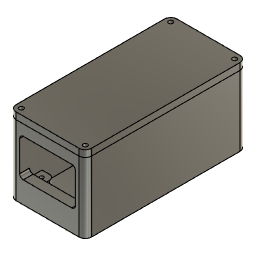
smarter-ac-unit (Autodesk Fusion 360 design; units mm, degrees)
Autodesk Fusion 360 part; units mm, degrees
sketch "top" plane through (0, 0, 0) normal (0, 0, 1) x (1, 0, 0)
  line L0 (0, 0) -> (31, 0)
  line L1 (31, 0) -> (31, 78.5)
  line L2 (31, 78.5) -> (0, 78.5)
  line L3 (0, 78.5) -> (0, 0)
  line L4 (36.5, -5.5) -> (36.5, 84)
  line L5 (36.5, 84) -> (-5.5, 84)
  line L6 (-5.5, 84) -> (-5.5, -5.5)
  line L7 (-5.5, -5.5) -> (36.5, -5.5)
  line L8 (-5.5, 39.25) -> (36.5, 39.25) construction
  line L9 (15.5, -5.5) -> (15.5, 84) construction
  line L10 (-5.5, -5.5) -> (0, 0) construction
  circle A0 centre (-2.2804, -2.2804) radius 1.225
  line L11 (-5.5, 67) -> (36.5, 67)
  line L12 (-5.5, 61.5) -> (0, 61.5)
  circle A1 centre (3.375, 3.375) radius 2.125
  circle A2 centre (3.375, 75.125) radius 2.125
  circle A3 centre (27.625, 3.375) radius 2.125
  circle A4 centre (27.625, 75.125) radius 2.125
  circle A5 centre (-2.2804, 80.7804) radius 1.225
  circle A6 centre (33.2804, -2.2804) radius 1.225
  circle A7 centre (33.2804, 80.7804) radius 1.225
  circle A8 centre (3.375, 3.375) radius 1
  circle A9 centre (27.625, 3.375) radius 1
  circle A10 centre (27.625, 75.125) radius 1
  circle A11 centre (3.375, 75.125) radius 1
  line L13 (0, 7) -> (7, 7)
  line L14 (7, 7) -> (7, 0)
  line L15 (24, 7) -> (24, 0)
  line L16 (31, 7) -> (24, 7)
  line L17 (24, 71.5) -> (24, 78.5)
  line L18 (31, 71.5) -> (24, 71.5)
  line L19 (7, 71.5) -> (7, 78.5)
  line L20 (0, 71.5) -> (7, 71.5)
  point P0 (-2.2804, -2.2804)
  dimension "d1" = 31
  dimension "d2" = 78.5
  dimension "d3" = 5.5
  dimension "d4" = 2.45
  dimension "d5" = 17
  dimension "d6" = 5.5
  dimension "d7" = 4.25
  dimension "d8" = 1.25
  dimension "d9" = 1.25
  dimension "d10" = 2
  dimension "d41" = 2
  dimension "d45" = 7
  dimension "d46" = 7
  constraint horizontal L0
  constraint vertical L1
  constraint horizontal L2
  constraint vertical L3
  constraint coincident L0.start L3.end
  constraint midpoint L6 L8.start
  constraint midpoint L4 L8.end
  constraint midpoint L7 L9.start
  constraint midpoint L5 L9.end
  constraint coincident P0 A0.centre
  constraint coincident L6 L11.start
  constraint coincident L4 L11.end
  constraint perpendicular L4 L11
  constraint coincident L6 L12.start
  constraint coincident L3 L12.end
  constraint perpendicular L3 L12
  constraint symmetric L8 A1 A2
  constraint symmetric L9 A1 A3
  constraint symmetric L9 A2 A4
  constraint coincident L10 P0
  constraint symmetric L8 A0 A5
  constraint symmetric L9 A0 A6
  constraint symmetric L9 A5 A7
  constraint concentric A1 A8
  constraint symmetric L9 A8 A9
  constraint symmetric L8 A8 A11
  constraint symmetric L8 A9 A10
  constraint coincident L3 L13.start
  constraint perpendicular L3 L13
  constraint coincident L0 L14.end
  constraint perpendicular L0 L14
  constraint symmetric L9 L13.start L16.start
  constraint symmetric L9 L13.end L15.start
  constraint symmetric L9 L14.end L15.end
  constraint symmetric L8 L13.start L20.start
  constraint symmetric L8 L13.end L19.start
  constraint symmetric L8 L14.end L19.end
  constraint symmetric L8 L15.start L17.start
  constraint symmetric L8 L15.end L17.end
  constraint symmetric L8 L16.start L18.start
  measures "d1" distance of L0.start L0.end
  measures "d2" distance of L0.start L2.end
  measures "d4" diameter of A0
  measures "d5" distance of L5 L11
  measures "d6" distance of L11 L12
  measures "d7" diameter of A1
  measures "d8" distance of L3 A1
  measures "d9" distance of L0 A1
  measures "d10" distance of L0.start A0
  measures "d41" diameter of A8
  measures "d45" distance of L13.start L13.end
  measures "d46" distance of L0 L13
extrude "Extrude1" add sketch "top" along normal blind 3 contours L0 L3 L13 L14 | L0 L1 L3 L4 L6 L7 L11 L12 | L0 L1 L3 L11 L13 L14 L15 L16 | L0 L1 L15 L16 | L3 L6 L11 L12 | L1 L2 L3 L4 L5 L6 L11 | L1 L2 L3 L11 L17 L18 L19 L20 | L2 L3 L19 L20 | L1 L2 L17 L18 | A0 | A1 | A2 | A3 | A4 | A5 | A6 | A7 | A8 | A9 | A10 | A11 makes body 1
extrude "Extrude2" add sketch "top" along normal blind 36 from surface at 3 contours L0 L1 L3 L4 L6 L7 L11 L12 | L3 L6 L11 L12 | L1 L2 L3 L4 L5 L6 L11 | A0 | A5 | A6 | A7 bodies 1
extrude "Extrude3" add sketch "top" along normal blind 6.5 from surface at 3 contours A1 | A2 | A3 | A4 | A8 | A9 | A10 | A11 bodies 1
sketch "side" plane through (-5.5, 0, 0) normal (-1, 0, 0) x (0, -1, 0)
  line L0 (-84, 0) -> (5.5, 0)
  line L1 (5.5, 0) -> (5.5, 39)
  line L2 (5.5, 39) -> (-84, 39)
  line L3 (-84, 39) -> (-84, 0)
  line L4 (-84, 0) -> (5.5, 0)
  line L5 (-84, 0) -> (-84, 39)
  line L6 (-84, 39) -> (5.5, 39)
  line L7 (5.5, 0) -> (5.5, 39)
  line L8 (-84, 19.5) -> (5.5, 19.5) construction
  line L9 (-1.25, 9.5) -> (-5.5, 9.5)
  line L10 (-73, 9.5) -> (-77.25, 9.5)
  line L11 (-5.5, 3) -> (-1.25, 3)
  line L12 (-77.25, 3) -> (-73, 3)
  line L13 (0, 3) -> (-78.5, 3)
  line L14 (0, 3) -> (0, 39)
  line L15 (-78.5, 3) -> (-78.5, 39)
  line L16 (-73, 9.5) -> (-5.5, 9.5) construction
  line L17 (-39.25, 39) -> (-39.25, 0) construction
  line L18 (-67, 0) -> (-67, 19.5) construction
  line L19 (-61.5, 0) -> (-61.5, 19.5) construction
  line L20 (-84, 14.5) -> (-61.5, 14.5) construction
  line L21 (-67, 14.5) -> (-61.5, 14.5)
  line L22 (-61.5, 14.5) -> (-61.5, 9.5)
  line L23 (-61.5, 9.5) -> (-67, 9.5)
  line L24 (-67, 9.5) -> (-67, 14.5)
  point P0 (-61.5, 0)
  point P1 (-67, 0)
  dimension "d19" = 5
  constraint midpoint L5 L8.start
  constraint midpoint L7 L8.end
  constraint coincident L10.start L16.start
  constraint coincident L9.end L16.end
  constraint midpoint L6 L17.start
  constraint midpoint L4 L17.end
  constraint coincident P1 L18.start
  constraint coincident L8 L18.end
  constraint perpendicular L8 L18
  constraint coincident P0 L19.start
  constraint coincident L8 L19.end
  constraint perpendicular L8 L19
  constraint coincident L5 L20.start
  constraint coincident L19 L20.end
  constraint perpendicular L19 L20
  constraint horizontal L21
  constraint vertical L22
  constraint horizontal L23
  constraint vertical L24
  constraint coincident L19 L22.end
  constraint coincident L16 L22.end
  constraint coincident L20 L21.start
  constraint coincident L18 L21.start
  measures "d19" distance of L16 L20
extrude "Extrude4" cut sketch "side" against normal up to surface (5.5 mm away) contours L21 L22 L23 L24 bodies 1
sketch "back" plane through (0, -5.5, 0) normal (0, -1, 0) x (1, 0, 0)
  line L0 (-5.5, 0) -> (36.5, 0)
  line L1 (36.5, 0) -> (36.5, 39)
  line L2 (36.5, 39) -> (-5.5, 39)
  line L3 (-5.5, 39) -> (-5.5, 0)
  line L4 (0, 3) -> (0, 39)
  line L5 (5.5, 9.5) -> (1.25, 9.5)
  line L6 (1.25, 3) -> (5.5, 3)
  line L7 (25.5, 3) -> (29.75, 3)
  line L8 (29.75, 9.5) -> (25.5, 9.5)
  line L9 (31, 3) -> (31, 39)
  line L10 (31, 3) -> (0, 3)
  line L11 (0, 39) -> (31, 39)
  line L12 (-5.5, 0) -> (36.5, 0)
  line L13 (36.5, 0) -> (36.5, 39)
  line L14 (-5.5, 0) -> (-5.5, 39)
  line L15 (0, 33) -> (31, 33)
  line L16 (0, 12) -> (31, 12)
  dimension "d22" = 6
  dimension "d23" = 2.5
  constraint coincident L4 L15.start
  constraint coincident L9 L15.end
  constraint perpendicular L9 L15
  constraint coincident L4 L16.start
  constraint coincident L9 L16.end
  constraint perpendicular L9 L16
  measures "d22" distance of L2 L15
  measures "d23" distance of L5 L16
extrude "Extrude5" cut sketch "back" against normal up to surface (5.5 mm away) contours L4 L9 L15 L16 bodies 1
sketch "front" plane through (0, 84, 0) normal (0, 1, 0) x (-1, 0, 0)
  line L0 (-36.5, 0) -> (5.5, 0)
  line L1 (5.5, 0) -> (5.5, 39)
  line L2 (5.5, 39) -> (-36.5, 39)
  line L3 (-36.5, 39) -> (-36.5, 0)
  line L4 (-36.5, 0) -> (-36.5, 39)
  line L5 (-36.5, 39) -> (5.5, 39)
  line L6 (5.5, 0) -> (5.5, 39)
  line L7 (-36.5, 0) -> (5.5, 0)
  line L8 (-25.5, 9.5) -> (-29.75, 9.5)
  line L9 (-1.25, 9.5) -> (-5.5, 9.5)
  line L10 (-31, 3) -> (0, 3)
  line L11 (0, 3) -> (0, 39)
  line L12 (-31, 3) -> (-31, 39)
  line L13 (-31, 12) -> (0, 12) construction
  line L14 (-15.5, 39) -> (-15.5, 12) construction
  circle A0 centre (-15.5, 12) radius 2.75
  dimension "d26" = 2.5
  dimension "d27" = 5.5
  constraint coincident L12 L13.start
  constraint coincident L11 L13.end
  constraint perpendicular L11 L13
  constraint midpoint L5 L14.start
  constraint midpoint L13 L14.end
  constraint coincident L14.end A0.centre
  measures "d26" distance of L8 L13
  measures "d27" diameter of A0
extrude "Extrude6" cut sketch "front" against normal up to surface (5.5 mm away) contours A0 bodies 1
extrude "Extrude7" cut sketch "top" against normal blind 5 from surface at 39 contours A0 | A5 | A6 | A7 bodies 1
sketch "lid" plane through (0, 0, 39) normal (0, 0, 1) x (-1, 0, 0)
  circle A0 centre (-33.2804, -80.7804) radius 1.225
  circle A1 centre (-33.2804, 2.2804) radius 1.225
  circle A2 centre (2.2804, -80.7804) radius 1.225
  circle A3 centre (2.2804, 2.2804) radius 1.225
  line L0 (-31, 0) -> (0, 0)
  line L1 (0, 0) -> (0, -78.5)
  line L2 (0, -78.5) -> (-31, -78.5)
  line L3 (-31, -78.5) -> (-31, 0)
  line L4 (5.5, -84) -> (5.5, 5.5)
  line L5 (5.5, 5.5) -> (-36.5, 5.5)
  line L6 (-36.5, 5.5) -> (-36.5, -84)
  line L7 (-36.5, -84) -> (5.5, -84)
  line L8 (5.5, -84) -> (5.5, 5.5)
  line L9 (-36.5, -84) -> (5.5, -84)
  line L10 (-36.5, 5.5) -> (-36.5, -84)
  line L11 (5.5, 5.5) -> (-36.5, 5.5)
  circle A4 centre (2.2804, 2.2804) radius 1.225
  circle A5 centre (-33.2804, 2.2804) radius 1.225
  circle A6 centre (-33.2804, -80.7804) radius 1.225
  circle A7 centre (2.2804, -80.7804) radius 1.225
  line L12 (0, 0) -> (0, -78.5)
  line L13 (0, -78.5) -> (-31, -78.5)
  line L14 (-31, -78.5) -> (-31, 0)
  line L15 (-31, 0) -> (0, 0)
extrude "Extrude8" add sketch "lid" along normal blind 3.75 separate body contours L0 L1 L2 L3 L12 L13 L14 L15 | L4 L5 L6 L7 L8 L9 L10 L11 makes body 2
fillet "Fillet1" radius 3.5 8 edges at (36.5, 84, 19.5) (-5.5, 84, 19.5) (-5.5, -5.5, 19.5) (36.5, -5.5, 19.5) (36.5, 84, 40.875) (-5.5, 84, 40.875) (-5.5, -5.5, 40.875) (36.5, -5.5, 40.875) on bodies 1 2
fillet "Fillet2" radius 2 4 edges at (31, -2.75, 33) (0, -2.75, 33) (0, -2.75, 12) (31, -2.75, 12) on bodies 1
fillet "Fillet3" radius 1.5 4 edges at (-2.75, 67, 14.5) (-2.75, 61.5, 14.5) (-2.75, 61.5, 9.5) (-2.75, 67, 9.5) on bodies 1
extrude "Extrude9" cut sketch "top" against normal blind 5 from surface at 9.5 contours A8 | A9 | A10 | A11 bodies 1
extrude "Extrude10" add sketch "top" along normal up to surface (6.5 mm away) from surface at 3 contours L0 L3 L13 L14 | L0 L1 L15 L16 | L2 L3 L19 L20 | L1 L2 L17 L18 bodies 1
fillet "Fillet4" radius 3 4 edges at (24, 71.5, 6.25) (24, 7, 6.25) (7, 7, 6.25) (7, 71.5, 6.25) on bodies 1
named bodies: "main", "lid"
